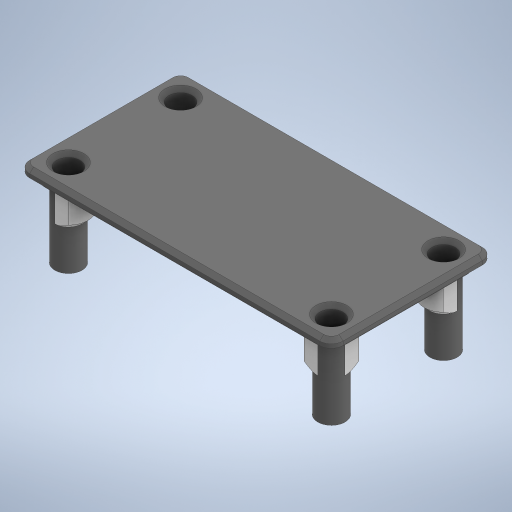
# Autodesk Inventor part: current_sensor_cover
Saved by Autodesk Inventor 2023 (Build 270158000, 158)
## iProperties
Created: 2023-10-27
Part Number: current_sensor_cover
Material: Generic
Document SubType Name: Modeling
Designer: mark
Density: 1 g/cm^3
Appearance: Default
Author: mark
Autodesk Inventor part; units mm, degrees
ref_plane "YZ Plane" through (0, 0, 0) normal (1, 0, 0) x (0, 1, 0)
ref_plane "XZ Plane" through (0, 0, 0) normal (0, 1, 0) x (-1, 0, 0)
ref_plane "XY Plane" through (0, 0, 0) normal (0, 0, 1) x (1, 0, 0)
sketch "Sketch1" plane through (0, 0, 0) normal (0, 1, 0) x (-1, 0, 0)
  line L0 (34.5, -18) -> (-34.5, -18)
  line L1 (-37.5, -15) -> (-37.5, 15)
  line L2 (-34.5, 18) -> (34.5, 18)
  line L3 (37.5, 15) -> (37.5, -15)
  line L4 (37.5, -21) -> (-37.5, -21)
  line L5 (-40.5, -18) -> (-40.5, 18)
  line L6 (-37.5, 21) -> (37.5, 21)
  line L7 (40.5, 18) -> (40.5, -18)
  arc A0 (37.5, -21) -> (40.5, -18) centre (37.5, -18) ccw
  arc A1 (34.5, -18) -> (37.5, -15) centre (34.5, -15) ccw
  arc A2 (37.5, 15) -> (34.5, 18) centre (34.5, 15) ccw
  arc A3 (40.5, 18) -> (37.5, 21) centre (37.5, 18) ccw
  arc A4 (-37.5, 21) -> (-40.5, 18) centre (-37.5, 18) ccw
  arc A5 (-34.5, 18) -> (-37.5, 15) centre (-34.5, 15) ccw
  arc A6 (-40.5, -18) -> (-37.5, -21) centre (-37.5, -18) ccw
  arc A7 (-37.5, -15) -> (-34.5, -18) centre (-34.5, -15) ccw
  line L8 (35, 19.5) -> (-35, 19.5)
  line L9 (-39, 15.5) -> (-39, -15.5)
  line L10 (-35, -19.5) -> (35, -19.5)
  line L11 (39, -15.5) -> (39, 15.5)
  arc A8 (39, 15.5) -> (35, 19.5) centre (35, 15.5) ccw
  arc A9 (-35, 19.5) -> (-39, 15.5) centre (-35, 15.5) ccw
  arc A10 (-39, -15.5) -> (-35, -19.5) centre (-35, -15.5) ccw
  arc A11 (35, -19.5) -> (39, -15.5) centre (35, -15.5) ccw
  point P0 (0, 0)
  point P1 (-37.5, 18)
  point P2 (-37.5, -18)
  point P3 (37.5, 18)
  dimension "d0" = 75
  dimension "d1" = 36
  dimension "d2" = 3
  dimension "d3" = 3
  dimension "d4" = 3
  dimension "d5" = 3
  dimension "d6" = 3
  dimension "d9" = 1.5
  dimension "d10" = 1.5
  dimension "d11" = 1.5
  dimension "d12" = 1.5
  dimension "d13" = 4
  dimension "d58" = 18
  dimension "d59" = 37.5
  constraints: 24 end point, 24 point on circle, 24 tangent, 12 centre point, 10 equal radius, 6 parallel, 6 point on line, 3 horizontal, 3 perpendicular
  measures "d0" distance of point (-37.5, 18) point (37.5, 18)
  measures "d1" distance of point (-37.5, -18) point (-37.5, 18)
  measures "d2" distance between parallel lines of L5 L1
  measures "d3" distance between parallel lines of L6 L2
  measures "d4" distance between parallel lines of L3 L7
  measures "d5" distance between parallel lines of L0 L4
  measures "d6" radius of A0
  measures "d9" distance between parallel lines of L2 L8
  measures "d10" distance between parallel lines of L11 L3
  measures "d11" distance between parallel lines of L10 L0
  measures "d12" distance between parallel lines of L1 L9
  measures "d13" radius of A8
  measures "d58" distance from line of point (0, 0) L0
  measures "d59" distance from line of L3 point (0, 0)
extrude "Extrusion1" add sketch "Sketch1" along normal blind 2 contours L0 A7 L1 A5 L2 A2 L3 A1 | L4 A6 L5 A4 L6 A3 L7 A0 | A8 L11 A11 L10 A10 L9 A9 L8
extrude "Extrusion2" add sketch "Sketch1" against normal blind 1.6 contours A8 L11 A11 L10 A10 L9 A9 L8
sketch "Sketch3" plane through (0, 2, 0) normal (0, 1, 0) x (1, 0, 0)
  line L0 (37.5, 21) -> (-37.5, 21) projected
  line L1 (-40.5, 18) -> (-40.5, -18) projected
  point P0 (0, 0)
  point P1 (-34, 14.5)
  dimension "d16" = 6.5
  dimension "d17" = 6.5
  measures "d16" distance from line of L0 point (-34, 14.5)
  measures "d17" distance from line of L1 point (-34, 14.5)
hole "Hole1" at (-34, 2, -14.5) direction (0, -1, 0) diameter 3.2 end through all
pattern_linear "Rectangular Pattern1" count 2 spacing 68 along (1, 0, 0) count 2 spacing 29 along (0, 0, 1) of "Hole1"
chamfer "Chamfer2" distance 1 angle 45 8 edges at (0, 2, -21) (-39.6213, 2, -20.1213) (-40.5, 2, 0) (-39.6213, 2, 20.1213) (0, 2, 21) (39.6213, 2, 20.1213) (40.5, 2, 0) (39.6213, 2, -20.1213)
sketch "Sketch4" plane through (0, 0, 0) normal (0, -1, 0) x (1, 0, 0)
  circle A0 centre (-34, 14.5) radius 1.6 projected
  circle A1 centre (-34, 14.5) radius 3.5
  circle A2 centre (34, 14.5) radius 1.6 projected
  circle A3 centre (34, 14.5) radius 3.5
  circle A4 centre (34, -14.5) radius 3.5
  circle A5 centre (-34, -14.5) radius 1.6 projected
  circle A6 centre (-34, -14.5) radius 3.5
  circle A7 centre (34, -14.5) radius 1.6
  circle A8 centre (34, -14.5) radius 1.6 projected
  point P0 (0, 0)
  dimension "d37" = 7
  dimension "d38" = 7
  dimension "d39" = 7
  dimension "d40" = 7
  constraints: 5 centre point, 5 coincident, 2 concentric
  measures "d37" diameter of A1
  measures "d38" diameter of A6
  measures "d39" diameter of A4
  measures "d40" diameter of A3
extrude "Extrusion3" add sketch "Sketch4" along normal blind 20.4
sketch "Sketch5" plane through (0, 2, 0) normal (0, 1, 0) x (1, 0, 0)
  circle A0 centre (34, -14.5) radius 1.6 projected
  circle A1 centre (34, -14.5) radius 3
  point P0 (0, 0)
  dimension "d43" = 6
  constraints: 1 centre point, 1 coincident
  measures "d43" diameter of A1
extrude "Extrusion4" cut sketch "Sketch5" against normal blind 10 contours A0 | A1
chamfer "Chamfer3" distance 1 angle 45 1 edges at (31, 2, 14.5)
pattern_linear "Rectangular Pattern2" count 2 spacing 29 along (0, 0, -1) count 2 spacing 68 along (-1, 0, 0) of "Extrusion4", "Chamfer3"
sketch "Sketch6" plane through (0, 0, 0) normal (0, -1, 0) x (1, 0, 0)
  circle A0 centre (-34, 14.5) radius 1.6 projected
  circle A1 centre (-34, 14.5) radius 5
  circle A2 centre (-34, 14.5) radius 3
  line L0 (-37.5, -14.5) -> (-37.5, 14.5) projected
  arc A3 (-37.5, 14.5) -> (-34, 18) centre (-34, 14.5) ccw projected
  line L1 (-37.5, 10.9293) -> (-37.5, 14.5)
  line L2 (34, 18) -> (-34, 18) projected
  line L3 (-30.4293, 18) -> (-34, 18)
  point P0 (0, 0)
  dimension "d55" = 10
  constraints: 4 end point, 2 centre point, 2 coincident, 2 point on circle, 2 point on line, 2 tangent, 1 collinear, 1 vertical
  measures "d55" diameter of A1
extrude "Extrusion5" add sketch "Sketch6" along normal blind 10 contours A1 L0 A3 L2 picked at (-33.6565, 10.0423)
mirror "Mirror1" about plane through (0, 0, 0) normal (0, 0, 1) of "Extrusion5"
mirror "Mirror2" about plane through (0, 0, 0) normal (1, 0, 0) of "Extrusion5", "Mirror1"
chamfer "Chamfer4" distance 1.5 angle 45 4 edges at (-30.4645, -10, -10.9645) (-30.4645, -10, 10.9645) (30.4645, -10, 10.9645) (30.4645, -10, -10.9645)
equation "\"d3\" = d2"
equation "\"d4\" = d2"
equation "\"d5\" = d2"
equation "\"d10\" = d9"
equation "\"d11\" = d9"
equation "\"d12\" = d9"
equation "\"d58\" = 0.5 * d1"
equation "\"d59\" = 0.5 * d0"
equation "\"d38\" = d37"
equation "\"d39\" = d38"
equation "\"d40\" = d37"
body "Solid1"
